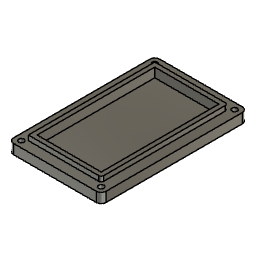
Smart Lock Enclosure Lid v2 (Autodesk Fusion 360 design; units mm, degrees)
Autodesk Fusion 360 part; units mm, degrees
sketch "Sketch1" plane through (0, 0, 0) normal (0, 0, 1) x (1, 0, 0)
  line L0 (47.5, 75) -> (-47.5, 75)
  line L1 (-47.5, 75) -> (-47.5, -75)
  line L2 (-47.5, -75) -> (47.5, -75)
  line L3 (47.5, -75) -> (47.5, 75)
  line L4 (47.5, 75) -> (-47.5, -75) construction
  line L5 (-47.5, 75) -> (47.5, -75) construction
  dimension "d1" = 95
  dimension "d2" = 150
  constraint horizontal L0
  constraint perpendicular L0 L1
  constraint parallel L0 L2
  constraint parallel L1 L3
  constraint coincident L4 origin
  constraint coincident L5 origin
  measures "d1" distance of L1.end L2.end
  measures "d2" distance of L0.end L1.end
extrude "Extrude1" add sketch "Sketch1" along normal blind 10
fillet "Fillet1" radius 5 1 edges at (47.5, -75, 5)
fillet "Fillet2" radius 5 1 edges at (47.5, 75, 5)
fillet "Fillet3" radius 5 1 edges at (-47.5, 75, 5)
fillet "Fillet4" radius 5 1 edges at (-47.5, -75, 5)
box "BoxPrimitive20" add length 129.8 width 74.8 height 5 placed x (0, -1, 0) y (1, 0, 0) z (0, 0, 1) at (-37.4, 64.9, 10)
fillet "Fillet12" radius 2.5 2 edges at (37.4, -64.9, 12.5) (37.4, 64.9, 12.5)
shell "Shell2" thickness 4.5 removed faces 1 at (-12.4667, -20.8, 15)
hole "Hole17" at (41, -68.5, 10) direction (0, 0, -1) diameter 5.5 depth 5 tip angle 180
hole "Hole18" at (-41, -68.5, 10) direction (0, 0, -1) diameter 5.5 depth 5 tip angle 180
hole "Hole19" at (-41, 68.5, 10) direction (0, 0, -1) diameter 5.5 depth 5 tip angle 180
hole "Hole20" at (41, 68.5, 10) direction (0, 0, -1) diameter 5.5 depth 5 tip angle 180
sketch "Sketch71" plane through (0, 0, 0) normal (0, 0, -1) x (1, 0, 0)
  arc A0 (-42.5, 75) -> (-47.5, 70) centre (-42.5, 70) ccw
  line L0 (-47.5, 70) -> (-47.5, -70)
  arc A1 (-47.5, -70) -> (-42.5, -75) centre (-42.5, -70) ccw
  line L1 (-42.5, -75) -> (42.5, -75)
  arc A2 (42.5, -75) -> (47.5, -70) centre (42.5, -70) ccw
  line L2 (47.5, -70) -> (47.5, 70)
  arc A3 (47.5, 70) -> (42.5, 75) centre (42.5, 70) ccw
  line L3 (42.5, 75) -> (-42.5, 75)
  line L4 (41.9268, 73.0838) -> (37.4937, 71.5945)
  line L5 (37.4937, 71.5945) -> (36.5669, 67.0107)
  line L6 (36.5669, 67.0107) -> (40.0732, 63.9162)
  line L7 (40.0732, 63.9162) -> (44.5063, 65.4055)
  line L8 (44.5063, 65.4055) -> (45.4331, 69.9893)
  line L9 (45.4331, 69.9893) -> (41.9268, 73.0838)
  line L10 (-45.5172, 69.7104) -> (-44.3068, 65.1932)
  line L11 (-44.3068, 65.1932) -> (-39.7896, 63.9828)
  line L12 (-39.7896, 63.9828) -> (-36.4828, 67.2896)
  line L13 (-36.4828, 67.2896) -> (-37.6932, 71.8068)
  line L14 (-37.6932, 71.8068) -> (-42.2104, 73.0172)
  line L15 (-42.2104, 73.0172) -> (-45.5172, 69.7104)
  line L16 (-36.598, -66.9213) -> (-40.1662, -63.8984)
  line L17 (-40.1662, -63.8984) -> (-44.5682, -65.4771)
  line L18 (-44.5682, -65.4771) -> (-45.402, -70.0787)
  line L19 (-45.402, -70.0787) -> (-41.8338, -73.1016)
  line L20 (-41.8338, -73.1016) -> (-37.4318, -71.5229)
  line L21 (-37.4318, -71.5229) -> (-36.598, -66.9213)
  line L22 (36.4225, -67.5425) -> (37.882, -71.9854)
  line L23 (37.882, -71.9854) -> (42.4595, -72.943)
  line L24 (42.4595, -72.943) -> (45.5775, -69.4575)
  line L25 (45.5775, -69.4575) -> (44.118, -65.0146)
  line L26 (44.118, -65.0146) -> (39.5405, -64.057)
  line L27 (39.5405, -64.057) -> (36.4225, -67.5425)
  point P0 (41, 68.5)
  point P1 (-41, 68.5)
  point P2 (-41, -68.5)
  point P3 (41, -68.5)
  dimension "d273" = 4.05
  dimension "d274" = 4.05
  dimension "d275" = 4.05
  dimension "d276" = 4.05
  measures "d273" distance of P0 L9
  measures "d274" distance of P1 L15
  measures "d275" distance of P2 L21
  measures "d276" distance of P3 L27
extrude "Extrude3" cut sketch "Sketch71" against normal blind 5 contours L4 L5 L6 L7 L8 L9 | L10 L11 L12 L13 L14 L15 | L16 L17 L18 L19 L20 L21 | L22 L23 L24 L25 L26 L27
